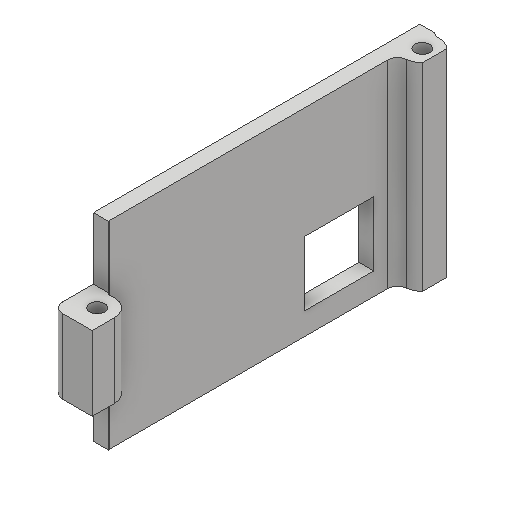
# Autodesk Inventor part: 3DP_PLA_Controller_Case_Side_Wall_Shorter
Saved by Autodesk Inventor 2026.1 (Build 301233000, 233)
## iProperties
Created: 2017-05-27
Part Number: 3DP_PLA_Controller_Case_Side_Wall_Shorter
Material: Ogólny
Document SubType Name: Modeling
Designer: Andrzej
Density: 1 g/cm^3
Appearance: Domyślna
Author: Andrzej
Autodesk Inventor part; units mm, degrees
ref_plane "YZ Plane" through (0, 0, 0) normal (1, 0, 0) x (0, 1, 0)
ref_plane "XZ Plane" through (0, 0, 0) normal (0, 1, 0) x (-1, 0, 0)
sketch "Szkic1" plane through (0, 0, 0) normal (0, 0, 1) x (1, 0, 0)
  circle A0 centre (-5.5, -12.5) radius 1.5
  circle A1 centre (-5.5, 53.1646) radius 1.5
  circle A2 centre (101.455, -12.5) radius 1.5
  arc A3 (-10, -15) -> (-8, -17) centre (-8, -15) ccw
  line L0 (-8, -17) -> (136.455, -17)
  arc A4 (136.455, -17) -> (141.455, -12) centre (136.455, -12) ccw
  line L1 (141.455, -12) -> (141.455, -2)
  arc A5 (141.455, -2) -> (136.455, 3) centre (136.455, -2) ccw
  line L2 (136.455, 3) -> (127.455, 3)
  arc A6 (115.455, 15) -> (127.455, 3) centre (127.455, 15) ccw
  line L3 (115.455, 15) -> (115.455, 29.1646)
  arc A7 (127.455, 41.1646) -> (115.455, 29.1646) centre (127.455, 29.1646) ccw
  line L4 (127.455, 41.1646) -> (136.455, 41.1646)
  arc A8 (136.455, 41.1646) -> (141.455, 46.1646) centre (136.455, 46.1646) ccw
  line L5 (141.455, 46.1646) -> (141.455, 56.1646)
  arc A9 (141.455, 56.1646) -> (136.455, 61.1646) centre (136.455, 56.1646) ccw
  line L6 (136.455, 61.1646) -> (122.455, 61.1646)
  line L7 (107.455, 76.1646) -> (122.455, 61.1646)
  line L8 (107.455, 76.1646) -> (107.455, 88.1646)
  arc A10 (107.455, 88.1646) -> (102.455, 93.1646) centre (102.455, 88.1646) ccw
  line L9 (102.455, 93.1646) -> (92.455, 93.1646)
  arc A11 (92.455, 93.1646) -> (87.455, 88.1646) centre (92.455, 88.1646) ccw
  line L10 (87.455, 88.1646) -> (87.455, 79.1646)
  arc A12 (75.455, 67.1646) -> (87.455, 79.1646) centre (75.455, 79.1646) ccw
  line L11 (75.455, 67.1646) -> (22, 67.1646)
  arc A13 (10, 79.1646) -> (22, 67.1646) centre (22, 79.1646) ccw
  line L12 (10, 79.1646) -> (10, 88.1646)
  arc A14 (10, 88.1646) -> (5, 93.1646) centre (5, 88.1646) ccw
  line L13 (5, 93.1646) -> (-5, 93.1646)
  arc A15 (-5, 93.1646) -> (-10, 88.1646) centre (-5, 88.1646) ccw
  line L14 (-10, 88.1646) -> (-10, -15)
  circle A16 centre (97.455, 83.1646) radius 2
  circle A17 centre (131.455, -7) radius 2
  circle A18 centre (131.455, 51.1646) radius 2
  circle A19 centre (0, 83.1646) radius 2
  line L15 (89.5711, 35.5361) -> (89.5711, 17.5361)
  arc A20 (83.5711, 11.5361) -> (89.5711, 17.5361) centre (83.5711, 17.5361) ccw
  line L16 (83.5711, 11.5361) -> (78.5711, 11.5361)
  arc A21 (72.5711, 17.5361) -> (78.5711, 11.5361) centre (78.5711, 17.5361) ccw
  line L17 (72.5711, 17.5361) -> (72.5711, 35.5361)
  arc A22 (78.5711, 41.5361) -> (72.5711, 35.5361) centre (78.5711, 35.5361) ccw
  line L18 (78.5711, 41.5361) -> (83.5711, 41.5361)
  arc A23 (89.5711, 35.5361) -> (83.5711, 41.5361) centre (83.5711, 35.5361) ccw
  line L19 (107.455, 22.1646) -> (107.455, 25.6646)
  line L20 (107.455, 25.6646) -> (109.455, 25.6646)
  line L21 (109.455, 25.6646) -> (109.455, 22.1646)
  line L22 (109.455, 22.1646) -> (107.455, 22.1646)
  line L23 (82.5, 60.1646) -> (86, 60.1646)
  line L24 (86, 60.1646) -> (86, 58.1646)
  line L25 (86, 58.1646) -> (82.5, 58.1646)
  line L26 (82.5, 58.1646) -> (82.5, 60.1646)
  line L27 (53.5, 60.1646) -> (57, 60.1646)
  line L28 (57, 60.1646) -> (57, 58.1646)
  line L29 (57, 58.1646) -> (53.5, 58.1646)
  line L30 (53.5, 58.1646) -> (53.5, 60.1646)
  line L31 (24.5, 60.1646) -> (28, 60.1646)
  line L32 (28, 60.1646) -> (28, 58.1646)
  line L33 (28, 58.1646) -> (24.5, 58.1646)
  line L34 (24.5, 58.1646) -> (24.5, 60.1646)
  line L35 (10, 58.1646) -> (10, 60.1646)
  line L36 (10, 60.1646) -> (13.5, 60.1646)
  line L37 (13.5, 60.1646) -> (13.5, 58.1646)
  line L38 (13.5, 58.1646) -> (10, 58.1646)
  line L39 (39, 60.1646) -> (42.5, 60.1646)
  line L40 (42.5, 60.1646) -> (42.5, 58.1646)
  line L41 (42.5, 58.1646) -> (39, 58.1646)
  line L42 (39, 58.1646) -> (39, 60.1646)
  line L43 (68, 60.1646) -> (71.5, 60.1646)
  line L44 (71.5, 60.1646) -> (71.5, 58.1646)
  line L45 (71.5, 58.1646) -> (68, 58.1646)
  line L46 (68, 58.1646) -> (68, 60.1646)
  line L47 (107.455, 37.6646) -> (107.455, 41.1646)
  line L48 (107.455, 41.1646) -> (109.455, 41.1646)
  line L49 (109.455, 41.1646) -> (109.455, 37.6646)
  line L50 (109.455, 37.6646) -> (107.455, 37.6646)
  line L51 (107.455, 6.6646) -> (107.455, 10.1646)
  line L52 (107.455, 10.1646) -> (109.455, 10.1646)
  line L53 (109.455, 10.1646) -> (109.455, 6.6646)
  line L54 (109.455, 6.6646) -> (107.455, 6.6646)
  line L55 (54.7961, 40.5361) -> (54.7961, 12.5361)
  arc A24 (48.7961, 6.5361) -> (54.7961, 12.5361) centre (48.7961, 12.5361) ccw
  line L56 (48.7961, 6.5361) -> (30.7961, 6.5361)
  arc A25 (24.7961, 12.5361) -> (30.7961, 6.5361) centre (30.7961, 12.5361) ccw
  line L57 (24.7961, 12.5361) -> (24.7961, 40.5361)
  arc A26 (30.7961, 46.5361) -> (24.7961, 40.5361) centre (30.7961, 40.5361) ccw
  line L58 (30.7961, 46.5361) -> (48.7961, 46.5361)
  arc A27 (54.7961, 40.5361) -> (48.7961, 46.5361) centre (48.7961, 40.5361) ccw
  circle A28 centre (65.8311, 7.4861) radius 1.6
  circle A29 centre (15.0311, 50.6661) radius 1.6
  circle A30 centre (89.9611, 50.6661) radius 1.6
  circle A31 centre (13.7611, 2.4061) radius 1.6
  circle A32 centre (65.8311, 35.4261) radius 1.6
  circle A33 centre (96.3111, 2.4061) radius 1.6
  line L59 (-7, 57.1646) -> (-7, -17)
  line L60 (-7, 57.1646) -> (-10, 57.1646)
  arc A34 (-7, 50.0023) -> (-7, 56.3269) centre (-5.5, 53.1646) ccw
  arc A35 (-7, -15.6623) -> (-7, -9.3377) centre (-5.5, -12.5) ccw
  line L61 (-2, -12.5) -> (-2, -17)
  point P0 (0, 0)
  point P1 (0, 0)
  dimension "d0" = 3
  dimension "d1" = 4
  dimension "d2" = 7
  dimension "d3" = 7
  dimension "d15" = 110.1646
  dimension "d16" = 65.6646
  constraints: 124 end point, 47 point on circle, 36 centre point, 7 point on line, 3 perpendicular, 2 coincident, 1 tangent
  measures "d0" distance between parallel lines of L14 L59
  measures "d1" distance from line of A1.centre L60
  measures "d2" diameter of A34
  measures "d3" diameter of A35
  measures "d15" distance between parallel lines of L13 L0
  measures "d16" distance of A0.centre A1.centre
extrude "Wyciągnięcie proste1" add sketch "Szkic1" along normal blind 40 contours L59 A35 | L59 L0 A3 L14 L60 | A35 L61 L0 L59 | L59 A34
sketch "Szkic3" plane through (0, 0, 0) normal (0, 0, -1) x (-1, 0, 0)
  line L0 (10, -8.75) -> (7, -8.75)
  circle A0 centre (5.5, -12.5) radius 1.5 projected
  circle A1 centre (5.5, 53.1646) radius 1.5 projected
  arc A2 (7, 56.3269) -> (7, 50.0023) centre (5.5, 53.1646) ccw projected
  line L1 (7, -9.3377) -> (7, 50.0023) projected
  arc A3 (7, -9.3377) -> (2, -12.5) centre (5.5, -12.5) ccw projected
  line L2 (2, -17) -> (2, -12.5) projected
  line L3 (8, -17) -> (2, -17) projected
  arc A4 (8, -17) -> (10, -15) centre (8, -15) ccw projected
  line L4 (10, 57.1646) -> (10, -15) projected
  line L5 (7, 57.1646) -> (10, 57.1646) projected
  line L6 (7, 56.3269) -> (7, 57.1646) projected
  point P0 (0, 0)
  dimension "d7" = 8.25
  constraints: 2 end point, 2 point on line, 1 horizontal
  measures "d7" distance between parallel lines of L3 L0
extrude "Wyciągnięcie proste2" cut sketch "Szkic3" against normal blind 12.5 contours L4 A4 L3 L2 A3 L1 L0
sketch "Szkic4" plane through (0, 0, 40) normal (0, 0, 1) x (1, 0, 0)
  circle A0 centre (-5.5, -12.5) radius 1.5 projected
  circle A1 centre (-5.5, 53.1646) radius 1.5 projected
  arc A2 (-7, 50.0023) -> (-7, 56.3269) centre (-5.5, 53.1646) ccw projected
  line L0 (-7, 56.3269) -> (-7, 57.1646) projected
  line L1 (-7, 57.1646) -> (-10, 57.1646) projected
  line L2 (-10, 57.1646) -> (-10, -15) projected
  arc A3 (-10, -15) -> (-8, -17) centre (-8, -15) ccw projected
  line L3 (-8, -17) -> (-2, -17) projected
  line L4 (-2, -17) -> (-2, -12.5) projected
  arc A4 (-2, -12.5) -> (-7, -9.3377) centre (-5.5, -12.5) ccw projected
  line L5 (-7, -9.3377) -> (-7, 50.0023) projected
  line L6 (-7, -8.75) -> (-10, -8.75) projected
  point P0 (0, 0)
extrude "Wyciągnięcie proste3" cut sketch "Szkic4" against normal blind 12.5 contours L5 A4 L4 L3 A3 L2 L6
fillet "Zaokrąglenie2" radius 2 2 edges at (-7, 56.3269, 20) (-7, 50.0023, 20)
fillet "Zaokrąglenie2" radius 0.6 1 edges at (-7, -9.3377, 20)
sketch "Szkic5" plane through (-10, 57.1646, 0) normal (-1, 0, 0) x (0, 0, 1)
  line L0 (27.5, -65.9146) -> (40, -65.9146) projected
  line L1 (40, 0) -> (40, -65.9146) projected
  line L2 (0, 0) -> (40, 0) projected
  line L3 (0, 0) -> (0, -65.9146) projected
  line L4 (0, -65.9146) -> (12.5, -65.9146) projected
  line L5 (12.5, -65.9146) -> (12.5, -72.1646) projected
  line L6 (12.5, -72.1646) -> (27.5, -72.1646) projected
  line L7 (27.5, -72.1646) -> (27.5, -65.9146) projected
  line L8 (17.5, -12.3) -> (4.5, -12.3)
  line L9 (4.5, -12.3) -> (4.5, -26.3)
  line L10 (4.5, -26.3) -> (17.5, -26.3)
  line L11 (17.5, -26.3) -> (17.5, -12.3)
  point P0 (0, -57.1646)
  dimension "d17" = 22.5
  dimension "d18" = 12.3
  dimension "d19" = 14
  dimension "d20" = 13
  constraints: 8 end point, 2 parallel, 1 horizontal, 1 perpendicular
  measures "d17" distance between parallel lines of L1 L11
  measures "d18" distance between parallel lines of L2 L8
  measures "d19" distance of L8.end L9.end
  measures "d20" distance between parallel lines of L9 L11
extrude "Wyciągnięcie proste4" cut sketch "Szkic5" against normal through all contours L11 L10 L9 L8
ref_plane "Płaszczyzna konstrukcyjna1" through (-2, 53.1646, 0) normal (1, 0, 0) x (0, 1, 0)
sketch "Szkic6" plane through (-2, 53.1646, 0) normal (1, 0, 0) x (0, 1, 0)
  line L0 (-8.6973, 46.9044) -> (25.5938, 46.9044)
  line L1 (25.5938, 46.9044) -> (25.5938, -6.7129)
  line L2 (25.5938, -6.7129) -> (-8.6973, -6.7129)
  line L3 (-8.6973, -6.7129) -> (-8.6973, 46.9044)
  point P0 (-53.1646, 0)
  constraints: 8 end point, 2 parallel, 1 horizontal, 1 perpendicular
extrude "Wyciągnięcie proste5" cut sketch "Szkic6" against normal blind 1
